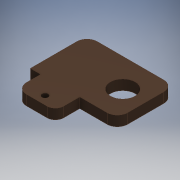
# Autodesk Inventor part: Верт. держатели
Saved by Autodesk Inventor 2018 (Build 220112000, 112)
## iProperties
Created: 2020-02-22
Part Number: Верт. держатели
Material: Типовые
Document SubType Name: Modeling
Designer: Leancher
Density: 1 g/cm^3
Appearance: По умолчанию
Author: Leancher
Autodesk Inventor part; units mm, degrees
ref_plane "YZ Plane" through (0, 0, 0) normal (1, 0, 0) x (0, 1, 0)
ref_plane "XZ Plane" through (0, 0, 0) normal (0, 1, 0) x (-1, 0, 0)
ref_plane "XY Plane" through (0, 0, 0) normal (0, 0, 1) x (1, 0, 0)
sketch "Эскиз1" plane through (0, 0, 0) normal (0, 0, 1) x (1, 0, 0)
  line L0 (-20, 5) -> (-20, 27.5449)
  arc A0 (22.2696, 27.5449) -> (17.2696, 32.5449) centre (17.2696, 27.5449) ccw
  line L1 (22.2696, 27.5449) -> (22.2696, 10)
  arc A1 (17.2696, 5) -> (22.2696, 10) centre (17.2696, 10) ccw
  circle A2 centre (-5, -2.85) radius 1.5
  line L2 (-15, 5) -> (-20, 5)
  line L3 (-15, 32.5449) -> (17.2696, 32.5449)
  arc A3 (-15, 32.5449) -> (-20, 27.5449) centre (-15, 27.5449) ccw
  line L4 (17.2696, 5) -> (4, 5)
  arc A4 (0, -6.85) -> (4, -2.85) centre (0, -2.85) ccw
  line L5 (4, -2.85) -> (4, 5)
  line L6 (0, -6.85) -> (-10, -6.85)
  line L7 (-15, -1.85) -> (-15, 5)
  arc A5 (-15, -1.85) -> (-10, -6.85) centre (-10, -1.85) ccw
  circle A6 centre (11.1348, 18.7724) radius 6
  point P0 (22.2696, 32.5449)
  point P1 (0, 32.5449)
  point P2 (22.2696, 5)
  dimension "d14" = 12
  dimension "d15" = 3
  constraints: 16 end point, 10 point on circle, 7 centre point
  measures "d14" diameter of A6
  measures "d15" diameter of A2
extrude "Выдавливание1" add sketch "Эскиз1" along normal blind 4.9
